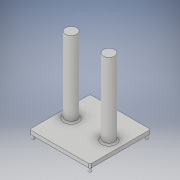
# Autodesk Inventor part: Final_mainstage
Saved by Autodesk Inventor 2019 (Build 230136000, 136)
## iProperties
Created: 2021-06-26
Part Number: Final_mainstage
Material: Generic
Document SubType Name: Modeling
Designer: 91742
Density: 1 g/cm^3
Appearance: Default
Author: 91742
Autodesk Inventor part; units mm, degrees
ref_plane "YZ Plane" through (0, 0, 0) normal (1, 0, 0) x (0, 1, 0)
ref_plane "XZ Plane" through (0, 0, 0) normal (0, 1, 0) x (-1, 0, 0)
ref_plane "XY Plane" through (0, 0, 0) normal (0, 0, 1) x (1, 0, 0)
sketch "Sketch1" plane through (0, 0, 0) normal (0, 1, 0) x (-1, 0, 0)
  line L0 (40, -40) -> (-40, -40)
  line L1 (-40, -40) -> (-40, 40)
  line L2 (-40, 40) -> (40, 40)
  line L3 (40, 40) -> (40, -40)
  line L4 (40, -40) -> (-40, 40) construction
  line L5 (-40, -40) -> (40, 40) construction
  line L6 (-40, 40) -> (-35, 40)
  line L7 (-40, 35) -> (-40, 40)
  line L8 (40, 40) -> (35, 40)
  line L9 (40, 35) -> (40, 40)
  line L10 (0, 0) -> (12.5837, 0)
  line L11 (-40, -40) -> (40, -40)
  line L12 (-40, -35) -> (-40, -40)
  line L13 (40, -40) -> (35, -40)
  circle A0 centre (37.5, 37.5) radius 2
  circle A1 centre (37.5, -37.5) radius 2
  circle A2 centre (-37.5, -37.5) radius 2
  circle A3 centre (-37.5, 37.5) radius 2
  dimension "d0" = 80
  dimension "d1" = 80
  dimension "d7" = 4
  dimension "d8" = 4
  dimension "d9" = 4
  constraints: 28 end point, 4 centre point, 4 horizontal, 2 midpoint, 2 parallel, 2 symmetric about line, 1 perpendicular
  measures "d0" distance of L1.end L2.end
  measures "d1" distance of L0.end L1.end
  measures "d7" diameter of A1
  measures "d8" diameter of A2
  measures "d9" diameter of A3
extrude "Extrusion1" add sketch "Sketch1" along normal blind 5
sketch "Sketch2" plane through (0, 0, 0) normal (0, -1, 0) x (1, 0, 0)
  point P0 (0, 0)
sketch "Sketch3" plane through (0, 0, 0) normal (0, -1, 0) x (1, 0, 0)
  line L0 (40, -40) -> (-40, -40)
  line L1 (-40, -40) -> (-40, 40)
  line L2 (-40, 40) -> (40, 40)
  line L3 (40, 40) -> (40, -40)
  line L4 (40, -40) -> (-40, 40) construction
  line L5 (-40, -40) -> (40, 40) construction
  line L6 (-40, 40) -> (-35, 40)
  line L7 (-40, 35) -> (-40, 40)
  line L8 (40, 40) -> (35, 40)
  line L9 (40, 35) -> (40, 40)
  line L10 (0, 0) -> (12.5837, 0)
  line L11 (40, -40) -> (35, -40)
  line L12 (-40, -40) -> (40, -40)
  line L13 (-40, -35) -> (-40, -40)
  circle A0 centre (37.5, 37.5) radius 2
  circle A1 centre (37.5, -37.5) radius 2
  circle A2 centre (-37.5, -37.5) radius 2
  circle A3 centre (-37.5, 37.5) radius 2
  dimension "d12" = 80
  dimension "d13" = 80
  dimension "d14" = 4
  dimension "d15" = 4
  dimension "d16" = 4
  constraints: 28 end point, 4 centre point, 4 horizontal, 2 midpoint, 2 parallel, 2 symmetric about line, 1 perpendicular
  measures "d12" distance of L2.start L9.end
  measures "d13" distance of L5.start L2.start
  measures "d14" diameter of A1
  measures "d15" diameter of A2
  measures "d16" diameter of A3
extrude "Extrusion2" add sketch "Sketch3" along normal mid plane 10 contours A0 | A1 | A2 | A3
sketch "Sketch4" plane through (0, 5, 0) normal (0, 1, 0) x (1, 0, 0)
  circle A0 centre (25, 0) radius 7.5
  circle A1 centre (-25, 0) radius 7.5
  point P0 (0, 0)
  dimension "d19" = 15
  dimension "d20" = 15
  constraints: 2 centre point
  measures "d19" diameter of A0
  measures "d20" diameter of A1
extrude "Extrusion3" add sketch "Sketch4" along normal blind 100
fillet "Fillet1" radius 2 6 edges at (-32.5, 5, 0) (17.5, 5, 0) (40, 2.5, 40) (-40, 2.5, 40) (-40, 2.5, -40) (40, 2.5, -40)
body "Solid1"
